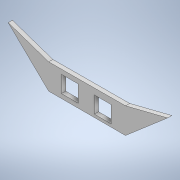
# Autodesk Inventor part: unwrappedDormerEastFacingPool
Saved by Autodesk Inventor 2020.1 (Build 241239000, 239)
## iProperties
Created: 2019-08-11
Part Number: unwrappedDormerEastFacingPool
Material: Generic
Document SubType Name: Modeling
Designer: steele
Density: 1 g/cm^3
Appearance: Default
Mass: 4.006e+06 g
Surface Area: 370938 cm^2
Volume: 4.006e+06 cm^3
Author: steele
Autodesk Inventor part; units mm, degrees
ref_plane "YZ Plane" through (0, 0, 0) normal (1, 0, 0) x (0, 1, 0)
ref_plane "XZ Plane" through (0, 0, 0) normal (0, 1, 0) x (-1, 0, 0)
ref_plane "XY Plane" through (0, 0, 0) normal (0, 0, 1) x (1, 0, 0)
sketch "Sketch1" plane through (0, 0, 0) normal (0, 0, 1) x (1, 0, 0)
  line L0 (-23.7527, 2860.8055) -> (2933.8428, 0)
  line L1 (2933.8428, 0) -> (2933.8428, 1854.2)
  line L2 (2933.8428, 0) -> (8547.2428, 0)
  line L3 (8547.2428, 0) -> (8547.2428, 1879.6)
  line L4 (2933.8428, 1854.2) -> (2933.8428, 0)
  line L5 (8547.2428, 0) -> (11626.9257, 2651.7257)
  line L6 (11626.9257, 2651.7257) -> (8547.2428, 1879.6)
  line L7 (3872.1661, 317.5) -> (5091.3661, 317.5)
  line L8 (5091.3661, 317.5) -> (5091.3661, 1536.7)
  line L9 (5091.3661, 1536.7) -> (3872.1661, 1536.7)
  line L10 (3872.1661, 1536.7) -> (3872.1661, 317.5)
  line L11 (3872.1661, 317.5) -> (5091.3661, 1536.7) construction
  line L12 (5091.3661, 317.5) -> (3872.1661, 1536.7) construction
  line L13 (-23.7527, 2860.8055) -> (2933.8428, 1854.2)
  line L14 (2933.8428, 1854.2) -> (8547.2428, 1879.6)
  line L15 (6275.5437, 213.6696) -> (7494.7437, 213.6696)
  line L16 (7494.7437, 213.6696) -> (7494.7437, 1432.8696)
  line L17 (7494.7437, 1432.8696) -> (6275.5437, 1432.8696)
  line L18 (6275.5437, 1432.8696) -> (6275.5437, 213.6696)
  line L19 (6275.5437, 213.6696) -> (7494.7437, 1432.8696) construction
  line L20 (7494.7437, 213.6696) -> (6275.5437, 1432.8696) construction
  point P0 (0, 0)
  point P1 (4481.7661, 927.1)
  point P2 (6885.1437, 823.2696)
  dimension "d2" = 5613.4
  dimension "d5" = 1219.2
  dimension "d6" = 1219.2
  dimension "d8" = 4114.8
  dimension "d11" = 1854.2
  dimension "d12" = 3124.2
  dimension "d13" = 1879.6
  dimension "d14" = 4064
  dimension "d15" = 3175
  dimension "d16" = 1219.2
  dimension "d17" = 1219.2
  constraints: 42 end point, 5 parallel, 4 midpoint, 3 horizontal, 3 perpendicular, 1 vertical
  measures "d2" distance of L0.end L2.end
  measures "d5" distance of L7.start L7.end
  measures "d6" distance of L8.end L7.end
  measures "d8" distance of L0.start L0.end
  measures "d11" distance of L0.end L1.end
  measures "d12" distance of L0.start L1.end
  measures "d13" distance of L2.end L3.end
  measures "d14" distance of L2.end L5.end
  measures "d15" distance of L5.end L3.end
  measures "d16" distance of L15.start L15.end
  measures "d17" distance of L16.end L15.end
extrude "Extrusion1" add sketch "Sketch1" against normal blind 304.8
body "Solid1"
